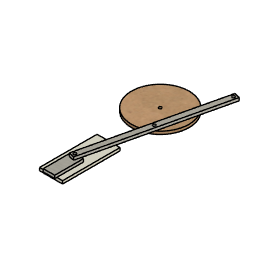
Elliptical drive (Autodesk Fusion 360 design; units mm, degrees)
Autodesk Fusion 360 part; units mm, degrees
sketch "Sketch1" plane through (0, 0, 0) normal (0, 0, 1) x (1, 0, 0) in component "Disk"
  circle A0 centre (0, 0) radius 50
  circle A1 centre (-45, 0) radius 2.5
  circle A2 centre (0, 0) radius 2.5
  dimension "d4" = 100
  dimension "d6" = 5
  dimension "d7" = 45
  dimension "d8" = 5
  constraint coincident A0.centre A2.centre
  measures "d4" diameter of A0
  measures "d6" diameter of A1
  measures "d7" distance of A0.centre A1.centre
  measures "d8" diameter of A2
extrude "Extrude1" add sketch "Sketch1" along normal blind 5 makes body 1 in component "Disk"
sketch "Sketch1 (2)" plane through (0, 0, 5) normal (0, 0, 1) x (-1, 0, 0) in component "Slider Block"
  circle A0 centre (45, 0) radius 2.5
  circle A1 centre (0, 0) radius 2.5
  circle A2 centre (0, 0) radius 50
  line L0 (115, -35) -> (95, -35)
  line L1 (95, -35) -> (95, 15)
  line L2 (95, 15) -> (115, 15)
  line L3 (115, 15) -> (115, -35)
  circle A3 centre (105, -30) radius 2.5
  dimension "d11" = 20
  dimension "d12" = 50
  dimension "d13" = 5
  dimension "d14" = 5
  constraint horizontal L0
  constraint vertical L1
  constraint horizontal L2
  constraint vertical L3
  measures "d11" distance of L0.start L0.end
  measures "d12" distance of L0.start L2.end
  measures "d13" diameter of A3
  measures "d14" distance of L0 A3.centre
extrude "Extrude1'" add sketch "Sketch1 (2)" against normal blind 5 separate body contours L0 L1 L2 L3 makes body 2 in component "Slider Block"
sketch "Sketch1 (3)" plane through (0, 0, 5) normal (0, 0, 1) x (-1, 0, 0) in component "Bar"
  circle A0 centre (45, 0) radius 2.5
  circle A1 centre (0, 0) radius 2.5
  circle A2 centre (0, 0) radius 50
  line L0 (-90, -50) -> (-100, -50)
  line L1 (-100, -50) -> (-100, 70)
  line L2 (-100, 70) -> (-90, 70)
  line L3 (-90, 70) -> (-90, -50)
  line L4 (-90, -50) -> (-100, -50)
  line L5 (-100, -50) -> (-100, -170)
  line L6 (-100, -170) -> (-90, -170)
  line L7 (-90, -170) -> (-90, -50)
  circle A3 centre (-95, -50) radius 2.5
  circle A4 centre (-95, -165) radius 2.5
  circle A5 centre (-95, 65) radius 2.5
  dimension "d17" = 120
  dimension "d18" = 10
  dimension "d19" = 120
  dimension "d20" = 5
  dimension "d23" = 5
  dimension "d24" = 5
  dimension "d25" = 5
  dimension "d26" = 5
  constraint horizontal L0
  constraint vertical L1
  constraint horizontal L2
  constraint vertical L3
  constraint horizontal L4
  constraint vertical L5
  constraint horizontal L6
  constraint vertical L7
  constraint midpoint L0 A3.centre
  measures "d17" distance of L0.start L2.end
  measures "d18" distance of L0.start L0.end
  measures "d19" distance of L0.start L6.end
  measures "d20" diameter of A3
  measures "d23" diameter of A4
  measures "d24" distance of L6 A4.centre
  measures "d25" diameter of A5
  measures "d26" distance of L2 A5.centre
extrude "Extrude2" add sketch "Sketch1 (3)" along normal blind 5 separate body contours L0 L4 L5 L6 L7 A3 | L0 L1 L2 L3 L4 A3 makes body 3 in component "Bar"
sketch "Sketch1 (4)" plane through (0, 0, 5) normal (0, 0, 1) x (-1, 0, 0) in component "Slider Base"
  circle A0 centre (45, 0) radius 2.5
  circle A1 centre (0, 0) radius 2.5
  circle A2 centre (0, 0) radius 50
  line L0 (20, 90) -> (-20, 90)
  line L1 (-20, 90) -> (-20, 190)
  line L2 (-20, 190) -> (20, 190)
  line L3 (20, 190) -> (20, 90)
  dimension "d41" = 40
  dimension "d42" = 100
  constraint horizontal L0
  constraint vertical L1
  constraint horizontal L2
  constraint vertical L3
  measures "d41" distance of L0.start L0.end
  measures "d42" distance of L0.start L2.end
extrude "Extrude1''" add sketch "Sketch1 (4)" along normal blind 5 separate body contours L0 L1 L2 L3 makes body 4 in component "Slider Base"
move_body "Move1" bodies 4 to x (1, 0, 0) y (0, 1, 0) z (0, 0, 1) at (0, 0, -10) in component "Slider Base"
component "Disk" placed x (0, 1, 0) y (-1, 0, 0) z (0, 0, 1) at (0, 0, 0)
component "Slider Block" placed x (-1, 0, 0) y (0, 1, 0) z (0, 0, -1) at (-105, -190, 5)
component "Bar" placed x (1, 0, 0) y (0, 1, 0) z (0, 0, 1) at (-95, -95, 0)
component "Slider Base" placed x (1, 0, 0) y (0, 1, 0) z (0, 0, 1) at (0, 0, 0)
equation "diskDiam = 100 mm"
equation "lengthA = 120 mm"
equation "lengthB = 120 mm"
equation "d4 = diskDiam"
equation "connectorDiam = 5 mm"
equation "d6 = connectorDiam"
equation "d7 = diskDiam / 2 - connectorDiam"
equation "d8 = connectorDiam"
equation "d13 = connectorDiam"
equation "d14 = connectorDiam"
equation "d17 = lengthA"
equation "d19 = lengthB"
equation "d20 = connectorDiam"
equation "d23 = connectorDiam"
equation "d25 = connectorDiam"
